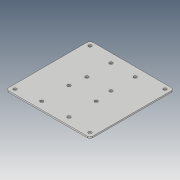
# Autodesk Inventor part: bottomPlate
Saved by Autodesk Inventor 2018 (Build 220112000, 112)
## iProperties
Created: 2020-02-01
Part Number: bottomPlate
Material: Generic
Document SubType Name: Modeling
Designer: anirudh
Density: 1 g/cm^3
Appearance: Default
Author: anirudh
Autodesk Inventor part; units mm, degrees
ref_plane "YZ Plane" through (0, 0, 0) normal (1, 0, 0) x (0, 1, 0)
ref_plane "XZ Plane" through (0, 0, 0) normal (0, 1, 0) x (-1, 0, 0)
ref_plane "XY Plane" through (0, 0, 0) normal (0, 0, 1) x (1, 0, 0)
sketch "Sketch1" plane through (0, 0, 0) normal (0, 1, 0) x (-1, 0, 0)
  line L0 (0, 0) -> (93.98, 0)
  line L1 (93.98, 0) -> (93.98, -93.98)
  line L2 (93.98, -93.98) -> (0, -93.98)
  line L3 (0, -93.98) -> (0, 0)
  line L4 (0, -93.98) -> (12.7, -93.98)
  line L5 (93.98, -93.98) -> (81.28, -93.98)
  line L6 (12.7, -93.98) -> (78.74, -93.98)
  line L7 (12.7, -93.98) -> (81.28, -93.98)
  arc A0 (33.54, -38.745) -> (29.94, -38.745) centre (31.74, -38.745) ccw
  circle A1 centre (31.74, -38.745) radius 1.8
  arc A2 (29.94, -8.245) -> (33.54, -8.245) centre (31.74, -8.245) ccw
  circle A3 centre (31.74, -8.245) radius 1.8
  arc A4 (64.04, -38.745) -> (60.44, -38.745) centre (62.24, -38.745) ccw
  circle A5 centre (62.24, -38.745) radius 1.8
  arc A6 (60.44, -8.245) -> (64.04, -8.245) centre (62.24, -8.245) ccw
  circle A7 centre (62.24, -8.245) radius 1.8
  line L8 (0, -93.98) -> (12.7, -93.98)
  line L9 (93.98, -93.98) -> (81.28, -93.98)
  line L10 (0, 0) -> (0, -46.99)
  line L11 (0, -46.99) -> (0, -93.98)
  circle A8 centre (60.49, -56.985) radius 1.75
  circle A9 centre (60.49, -83.985) radius 1.75
  circle A10 centre (33.49, -56.985) radius 1.75
  circle A11 centre (33.49, -83.985) radius 1.75
  constraints: 24 end point, 8 centre point, 8 point on circle, 4 coincident, 4 horizontal alignment, 3 collinear, 2 horizontal, 2 parallel, 2 point on line, 1 midpoint, 1 perpendicular, 8 other
extrude "Extrusion5" add sketch "Sketch1" along normal blind 1.5875
fillet "Fillet2" radius 3.175 4 edges at (0, 0.7937, 0) (0, 0.7937, -93.98) (-93.98, 0.7937, 0) (-93.98, 0.7937, -93.98)
sketch "Sketch4" plane through (0, 1.5875, 0) normal (0, 1, 0) x (1, 0, 0)
  line L0 (-3.175, 93.98) -> (-90.805, 93.98) projected
  circle A0 centre (-88.9, 5.08) radius 1.75
  circle A1 centre (-88.9, 88.9) radius 1.75
  circle A2 centre (-5.08, 5.08) radius 1.75
  circle A3 centre (-5.08, 88.9) radius 1.75
  point P0 (0, 0)
  dimension "d37" = 3.5
  dimension "d38" = 3.5
  dimension "d39" = 3.5
  dimension "d40" = 3.5
  constraints: 4 centre point
  measures "d37" diameter of A0
  measures "d38" diameter of A1
  measures "d39" diameter of A2
  measures "d40" diameter of A3
extrude "Extrusion6" cut sketch "Sketch4" against normal blind 1.5875
body "Solid2"
